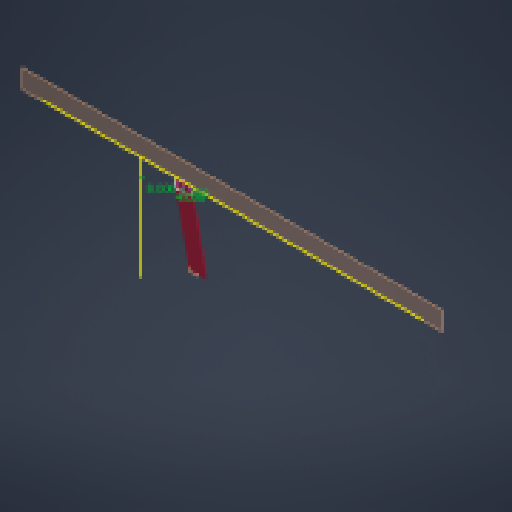
# Autodesk Inventor part: Bottom jaw diagonals 2
Saved by Autodesk Inventor 2027 (Build 310192000, 192)
## iProperties
Created: 2026-05-26
Part Number: Bottom jaw diagonals 2
Material: Generic
Document SubType Name: Modeling
Designer: lucas
Density: 1 g/cm^3
Appearance: Default
Author: lucas
Autodesk Inventor part; units mm, degrees
ref_plane "YZ Plane" through (0, 0, 0) normal (1, 0, 0) x (0, 1, 0)
ref_plane "XZ Plane" through (0, 0, 0) normal (0, 1, 0) x (-1, 0, 0)
ref_plane "XY Plane" through (0, 0, 0) normal (0, 0, 1) x (1, 0, 0)
ref_plane "Work Plane1" through (0, 0, 0) normal (0, 0, 1) x (1, 0, 0)
sketch "Sketch1" plane through (0, 0, 0) normal (0, 0, 1) x (1, 0, 0)
  line L0 (0, -101.6) -> (101.6, -101.6)
  line L1 (101.6, -101.6) -> (101.6, -50.8)
  line L2 (101.6, -50.8) -> (0, -50.8)
  line L3 (0, -50.8) -> (0, -101.6)
  point P0 (0, 0)
  point P1 (50.8, -76.2)
  dimension "d0" = 101.6
  dimension "d1" = 50.8
  constraints: 8 end point, 2 parallel, 1 horizontal, 1 perpendicular, 1 other
  measures "d0" distance of L0.start L0.end
  measures "d1" distance of L2.end L0.start
ref_plane "Work Plane3" through (533.4, 660.4, 279.4) normal (0, 0, 1) x (1, 0, 0)
sketch "Sketch3" plane through (533.4, 660.4, 279.4) normal (0, 0, 1) x (1, 0, 0)
  line L0 (1117.6, -50.8) -> (-1117.6, -50.8) projected
  line L1 (-533.4, -50.8) -> (-533.4, -660.4) projected
  line L2 (-228.6, -50.8) -> (-330.2, -50.8)
  line L3 (-330.2, -50.8) -> (-330.2, -101.6)
  line L4 (-330.2, -101.6) -> (-228.6, -101.6)
  line L5 (-228.6, -101.6) -> (-228.6, -50.8)
  point P0 (-279.4, -76.2)
  dimension "d16" = 101.6
  dimension "d17" = 50.8
  dimension "d18" = 203.2
  constraints: 8 end point, 2 parallel, 1 horizontal, 1 perpendicular, 1 point on line
  measures "d16" distance of L3.end L4.end
  measures "d17" distance of L4.end L2.start
  measures "d18" distance from line of L1 L3.end
sketch3d "3D Sketch4"
  line L0 (50.8, -76.2, 0) -> (254, 584.2, 279.4)
sweep "Sweep2" add profiles "Sketch1" path "3D Sketch4"
body "Solid2"
